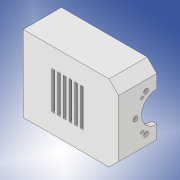
# Autodesk Inventor part: FA002
Saved by Autodesk Inventor 2017 SP1 (Build 210196100, 196)
## iProperties
Created: 2017-06-16
Part Number: FA002
Material: ABS Plastic
Document SubType Name: Modeling
Designer: Zach
Density: 1.06 g/cm^3
Appearance: CR White
Author: Zach
Autodesk Inventor part; units mm, degrees
ref_plane "YZ Plane" through (0, 0, 0) normal (1, 0, 0) x (0, 1, 0)
ref_plane "XZ Plane" through (0, 0, 0) normal (0, 1, 0) x (-1, 0, 0)
ref_plane "XY Plane" through (0, 0, 0) normal (0, 0, 1) x (1, 0, 0)
sketch "Sketch1" plane through (0, 0, 0) normal (0, 0, 1) x (1, 0, 0)
  line L0 (0, 0) -> (100, 0)
  line L1 (100, 0) -> (100, 80) construction
  line L2 (100, 80) -> (0, 80)
  line L3 (0, 80) -> (0, 0)
  line L4 (100, 70) -> (90, 80)
  line L5 (100, 10) -> (90, 0)
  line L6 (100, 70) -> (100, 10)
  dimension "d0" = 100
  dimension "d1" = 80
  dimension "d23" = 10
  dimension "d24" = 10
  dimension "d25" = 10
  dimension "d26" = 10
  constraints: 14 end point, 4 point on line, 2 parallel, 2 perpendicular, 1 horizontal
  measures "d0" distance of L2.end L1.end
  measures "d1" distance of L1.end L0.end
  measures "d23" distance of L1.end L4.end
  measures "d24" distance of L1.end L4.start
  measures "d25" distance of L0.end L5.start
  measures "d26" distance of L5.end L0.end
extrude "Extrusion1" add sketch "Sketch1" along normal blind 40
sketch "Sketch4" plane through (0, 0, 0) normal (0, 0, -1) x (-1, 0, 0)
  line L0 (-90, 80) -> (0, 80) projected
  line L1 (0, 0) -> (-90, 0) projected
  line L2 (-100, 70) -> (-90, 80) projected
  line L3 (-100, 10) -> (-100, 70) projected
  line L4 (-90, 0) -> (-100, 10) projected
  line L5 (0, 75) -> (-87.9289, 75)
  line L6 (-87.9289, 75) -> (-95, 67.9289)
  line L7 (-95, 67.9289) -> (-95, 12.0711)
  line L8 (-95, 12.0711) -> (-87.9289, 5)
  line L9 (-87.9289, 5) -> (0, 5)
  line L10 (0, 75) -> (0, 5)
  line L11 (0, 80) -> (0, 0) projected
  dimension "d27" = 5
  constraints: 12 end point, 1 collinear, 4 other
  measures "d27" distance between parallel lines of L0 L5
extrude "Extrusion4" cut sketch "Sketch4" against normal blind 35 contours L10 L9 L8 L7 L6 L5
sketch "Sketch5" plane through (0, 0, 40) normal (-1, 0, 0) x (0, 0, 1)
  line L0 (0, 0) -> (0, 80)
  line L1 (-40, 5) -> (-40, 75)
  line L2 (0, 80) -> (-40, 80)
  line L3 (-40, 80) -> (-40, 70)
  line L4 (-40, 70) -> (0, 70)
  line L5 (0, 70) -> (0, 80)
  line L6 (0, 80) -> (-10, 80)
  line L7 (-10, 80) -> (-10, 50)
  line L8 (-10, 50) -> (0, 50)
  line L9 (0, 50) -> (0, 80)
  line L10 (-40, 0) -> (0, 0)
  dimension "d15" = 10
  dimension "d16" = 10
  dimension "d17" = 50
  constraints: 22 end point, 4 parallel, 2 horizontal, 2 perpendicular, 1 coincident, 1 point on line
  measures "d15" distance of L3.end L2.end
  measures "d16" distance of L8.end L7.end
  measures "d17" distance between parallel lines of L10 L8
extrude "Extrusion5" add sketch "Sketch5" against normal blind 5
sketch "Sketch6" plane through (100, 10, 0) normal (1, 0, 0) x (0, 0, -1)
  circle A0 centre (0, 30) radius 16
  line L0 (0, 0) -> (0, 60) projected
  dimension "d20" = 32
  constraints: 1 centre point, 1 coincident, 1 midpoint
  measures "d20" diameter of A0
extrude "Extrusion6" cut sketch "Sketch6" against normal through all
sketch "Sketch7" plane through (0, 0, 35) normal (0, 0, -1) x (-1, 0, 0)
  line L0 (-87.9289, 75) -> (-5, 75) projected
  line L1 (0, 5) -> (-87.9289, 5) projected
  line L2 (-74, 75) -> (-69, 75)
  line L3 (-69, 75) -> (-69, 5)
  line L4 (-69, 5) -> (-74, 5)
  line L5 (-74, 5) -> (-74, 75)
  line L6 (-95, 56) -> (-95, 67.9289) projected
  line L7 (-24, 75) -> (-19, 75)
  line L8 (-19, 75) -> (-19, 5)
  line L9 (-19, 5) -> (-24, 5)
  line L10 (-24, 5) -> (-24, 75)
  line L11 (-69, 67.5) -> (-24, 67.5)
  line L12 (-24, 67.5) -> (-24, 62.5)
  line L13 (-24, 62.5) -> (-69, 62.5)
  line L14 (-69, 62.5) -> (-69, 67.5)
  line L15 (-69, 17.5) -> (-24, 17.5)
  line L16 (-24, 17.5) -> (-24, 12.5)
  line L17 (-24, 12.5) -> (-69, 12.5)
  line L18 (-69, 12.5) -> (-69, 17.5)
  line L19 (-46.5, 67.5) -> (-46.5, 12.5) construction
  point P0 (0, 0)
  point P1 (-46.5, 40)
  point P2 (-69, 40)
  dimension "d28" = 5
  dimension "d29" = 21
  dimension "d30" = 5
  dimension "d31" = 45
  dimension "d32" = 5
  dimension "d33" = 5
  dimension "d34" = 45
  constraints: 34 end point, 8 parallel, 8 point on line, 4 horizontal, 4 midpoint, 4 perpendicular, 1 horizontal alignment
  measures "d28" distance between parallel lines of L3 L5
  measures "d29" distance between parallel lines of L6 L5
  measures "d30" distance between parallel lines of L8 L10
  measures "d31" distance between parallel lines of L3 L10
  measures "d32" distance between parallel lines of L13 L11
  measures "d33" distance between parallel lines of L15 L17
  measures "d34" distance between parallel lines of L15 L13
extrude "Extrusion7" add sketch "Sketch7" along normal blind 35 contours L0 L3 L1 L5 | L0 L8 L1 L10 | L11 L10 L13 L3 | L3 L15 L10 L17
sketch "Sketch8" plane through (0, 0, 0) normal (0, 0, -1) x (-1, 0, 0)
  line L0 (-19, 5) -> (-19, 75) projected
  line L1 (-69, 17.5) -> (-24, 17.5) projected
  line L2 (-19, 5) -> (-42, 5)
  line L3 (-42, 5) -> (-42, 17.5)
  line L4 (-42, 17.5) -> (-19, 17.5)
  line L5 (-19, 17.5) -> (-19, 5)
  point P0 (0, 0)
  dimension "d37" = 23
  constraints: 8 end point, 2 parallel, 1 horizontal, 1 perpendicular, 1 point on line
  measures "d37" distance of L3.end L4.end
extrude "Extrusion8" cut sketch "Sketch8" against normal blind 10
sketch "Sketch9" plane through (69, 17.5, 35) normal (-1, 0, 0) x (0, 0, 1)
  line L0 (-35, 0) -> (-35, 45) projected
  circle A0 centre (-35, 22.5) radius 2.75
  line L1 (-50.5, 7) -> (-19.5, 7) construction
  line L2 (-19.5, 7) -> (-19.5, 38) construction
  line L3 (-19.5, 38) -> (-50.5, 38) construction
  line L4 (-50.5, 38) -> (-50.5, 7) construction
  line L5 (-50.5, 7) -> (-19.5, 38) construction
  line L6 (-19.5, 7) -> (-50.5, 38) construction
  circle A1 centre (-19.5, 38) radius 1.5
  circle A2 centre (-19.5, 7) radius 1.5
  point P0 (-35, -17.5)
  dimension "d40" = 5.5
  dimension "d41" = 31
  dimension "d42" = 31
  dimension "d43" = 3
  dimension "d44" = 3
  constraints: 12 end point, 3 centre point, 3 midpoint, 2 coincident, 2 parallel, 1 horizontal, 1 perpendicular
  measures "d40" diameter of A0
  measures "d41" distance of L3.end L2.end
  measures "d42" distance of L2.end L1.end
  measures "d43" diameter of A1
  measures "d44" diameter of A2
extrude "Extrusion9" cut sketch "Sketch9" against normal through all
sketch "Sketch10" plane through (0, 0, 35) normal (0, 0, -1) x (-1, 0, 0)
  line L0 (-30, 59.5) -> (-33, 59.5)
  line L1 (-33, 59.5) -> (-33, 20.5)
  line L2 (-33, 20.5) -> (-30, 20.5)
  line L3 (-30, 20.5) -> (-30, 59.5)
  line L4 (-24, 62.5) -> (-24, 17.5) projected
  line L5 (-69, 62.5) -> (-24, 62.5) projected
  line L6 (-24, 17.5) -> (-19, 17.5) projected
  line L7 (-36, 59.5) -> (-39, 59.5)
  line L8 (-39, 59.5) -> (-39, 20.5)
  line L9 (-39, 20.5) -> (-36, 20.5)
  line L10 (-36, 20.5) -> (-36, 59.5)
  line L11 (-42, 59.5) -> (-45, 59.5)
  line L12 (-45, 59.5) -> (-45, 20.5)
  line L13 (-45, 20.5) -> (-42, 20.5)
  line L14 (-42, 20.5) -> (-42, 59.5)
  line L15 (-48, 59.5) -> (-51, 59.5)
  line L16 (-51, 59.5) -> (-51, 20.5)
  line L17 (-51, 20.5) -> (-48, 20.5)
  line L18 (-48, 20.5) -> (-48, 59.5)
  line L19 (-54, 59.5) -> (-57, 59.5)
  line L20 (-57, 59.5) -> (-57, 20.5)
  line L21 (-57, 20.5) -> (-54, 20.5)
  line L22 (-54, 20.5) -> (-54, 59.5)
  line L23 (-60, 59.5) -> (-63, 59.5)
  line L24 (-63, 59.5) -> (-63, 20.5)
  line L25 (-63, 20.5) -> (-60, 20.5)
  line L26 (-60, 20.5) -> (-60, 59.5)
  point P0 (0, 0)
  dimension "d47" = 3
  dimension "d49" = 6
  dimension "d50" = 3
  dimension "d51" = 3
  dimension "d54" = 6
  constraints: 48 end point, 2 horizontal, 2 parallel, 1 perpendicular, 40 other
  measures "d47" distance of L2.end L1.end
  measures "d49" distance between parallel lines of L4 L3
  measures "d50" distance from line of L5 L0.start
  measures "d51" distance between parallel lines of L6 L2
  measures "d54" distance of L0.start L7.start
extrude "Extrusion10" cut sketch "Sketch10" against normal through all
sketch "Sketch11" plane through (0, 0, 0) normal (0, -1, 0) x (1, 0, 0)
  circle A0 centre (45, 0) radius 6
  line L0 (0, 0) -> (90, 0) projected
  dimension "d61" = 12
  constraints: 1 centre point, 1 coincident, 1 midpoint
  measures "d61" diameter of A0
extrude "Extrusion11" cut sketch "Sketch11" against normal blind 5
sketch "Sketch12" plane through (69, 17.5, 35) normal (-1, 0, 0) x (0, 0, 1)
  arc A0 (-35, 19.75) -> (-35, 25.25) centre (-35, 22.5) ccw projected
  circle A1 centre (-35, 22.5) radius 12.5
  point P0 (-35, -17.5)
  dimension "d64" = 25
  constraints: 1 centre point, 1 coincident
  measures "d64" diameter of A1
extrude "Extrusion12" cut sketch "Sketch12" against normal blind 2
sketch "Sketch13" plane through (100, 10, 40) normal (1, 0, 0) x (0, 0, -1)
  arc A0 (40, 46) -> (40, 14) centre (40, 30) ccw projected
  circle A1 centre (17.5, 30) radius 2.5
  circle A2 centre (28.75, 10.5144) radius 2.5
  circle A3 centre (51.25, 10.5144) radius 2.5
  circle A4 centre (62.5, 30) radius 2.5
  circle A5 centre (51.25, 49.4856) radius 2.5
  circle A6 centre (28.75, 49.4856) radius 2.5
  point P0 (40, -10)
  dimension "d67" = 5
  dimension "d68" = 22.5
  dimension "d71" = 360
  constraints: 6 centre point, 1 horizontal alignment, 13 other
  measures "d67" diameter of A1
  measures "d68" distance of A1.centre A0.centre
extrude "Extrusion13" cut sketch "Sketch13" against normal blind 10 contours A1 | A2 | A6
body "Solid1"
